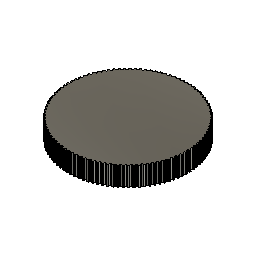
gear_99z (Autodesk Fusion 360 design; units mm, degrees)
Autodesk Fusion 360 part; units mm, degrees
sketch "Sketch1" plane through (0, 0, 0) normal (0, 0, 1) x (1, 0, 0) in component "gt2 pulley"
  circle A0 centre (0, 0) radius 31.5127 construction
  circle A1 centre (0, 0) radius 30.5087 construction
  line L0 (0, 0) -> (0, 31.5127) construction
  line L1 (0, 0) -> (0.9998, 31.4968) construction
  line L2 (0, 0) -> (1.4041, 31.4814) construction
  circle A2 centre (0, 0) radius 31.2587 construction
  arc A3 (0.3982, 31.1233) -> (0.4778, 30.824) centre (1.3927, 31.2276) ccw
  circle A4 centre (0, 0) radius 31.1087 construction
  arc A5 (0.2501, 31.2577) -> (0, 31.2587) centre (0, 0) ccw
  arc A6 (0.3982, 31.1233) -> (0.2501, 31.2577) centre (0.249, 31.1077) ccw
  arc A7 (0.4778, 30.824) -> (0.968, 30.4933) centre (0.9856, 31.048) ccw
  arc A8 (0, 31.2587) -> (-0.2501, 31.2577) centre (0, 0) ccw
  arc A9 (-0.2501, 31.2577) -> (-0.3982, 31.1233) centre (-0.249, 31.1077) ccw
  arc A10 (-0.4778, 30.824) -> (-0.3982, 31.1233) centre (-1.3927, 31.2276) ccw
  arc A11 (-0.9678, 30.4933) -> (-0.4778, 30.824) centre (-0.9856, 31.048) ccw
  arc A12 (0.968, 30.4933) -> (-0.968, 30.4933) centre (0, 0) ccw
  point P0 (1.3927, 31.2276)
  point P1 (0, 31.2587)
  dimension "d18" = 63.0254
  dimension "d19" = 1.818
  dimension "d22" = 1.004
  dimension "d24" = 0.75
  dimension "d26" = 1
  dimension "d27" = 0.15
  dimension "d28" = 0.15
  dimension "d47" = 0.555
  dimension "d52" = 3.812
  constraint coincident A0.centre A1.centre
  constraint coincident A0 L0.end
  constraint vertical L0
  constraint coincident A0 L1.end
  constraint coincident A0 L2.end
  constraint concentric A1 A2
  constraint coincident A1 A7.end
  constraint coincident L1 A7.end
  constraint coincident A2 P0
  constraint coincident L2 P0
  constraint coincident P0 A3.centre
  constraint coincident A2 P1
  constraint coincident L0 P1
  constraint concentric A2 A4
  constraint coincident P1 A5.end
  constraint coincident A4 A6.centre
  constraint coincident A3.start A6.start
  constraint tangent A3 A6
  constraint tangent A3 A7
  constraint symmetric L0 A7.end A12.end
  constraint symmetric L0 A3.start A9.end
  constraint symmetric L0 A3.end A10.start
  constraint symmetric L0 A3 A10
  constraint symmetric L0 A5.start A8.end
  constraint symmetric L0 P1 A5.end
  constraint symmetric L0 A5 A8
  constraint symmetric L0 A6 A9
  constraint symmetric L0 A7 A11
  constraint coincident A1 A11.start
  constraint tangent A1 A7
  constraint coincident L1 A7.centre
  measures "d18" diameter of A0
  measures "d19" angle of L0 L1
  measures "d22" distance of A0 A1
  measures "d24" distance of A1 A2
  measures "d26" radius of A3
  measures "d27" distance of A2 A4
  measures "d28" radius of A6
  measures "d47" radius of A7
extrude "Extrude1" add sketch "Sketch1" along normal blind 10 makes body 1
pattern_circular "C-Pattern1" count 99 over 360 about axis through (0, 0, 1.75) along (0, 0, 1) of bodies 1 makes body 2 at (-2.0422, 30.4402, 6.6667) makes body 3 at (-3.1141, 30.3493, 3.3333) makes body 4 at (-5.0327, 30.0907, 3.3333) makes body 5 at (-6.9311, 29.7109, 3.3333) makes body 6 at (-10.232, 28.7417, 6.6667) makes body 7 at (-11.4386, 28.2832, 6.6667) makes body 8 at (-13.7882, 27.2152, 6.6667) makes body 9 at (-14.1707, 27.0179, 3.3333) makes body 10 at (-17.1225, 25.2507, 6.6667) makes body 11 at (-17.477, 25.0067, 3.3333) makes body 12 at (-19.0278, 23.8479, 3.3333) makes body 13 at (-21.5918, 21.554, 6.6667) makes body 14 at (-21.8937, 21.2472, 6.6667) makes body 15 at (-23.1972, 19.8159, 3.3333) makes body 16 at (-24.9138, 17.6091, 6.6667) makes body 17 at (-26.2035, 15.6256, 6.6667) makes body 18 at (-26.5282, 15.0677, 3.3333) makes body 19 at (-27.7961, 12.5759, 6.6667) makes body 20 at (-28.5378, 10.7877, 6.6667) makes body 21 at (-28.9004, 9.7749, 3.3333) makes body 22 at (-29.4621, 7.9222, 3.3333) makes body 23 at (-30.0637, 5.1919, 6.6667) makes body 24 at (-30.3324, 3.2747, 6.6667) makes body 25 at (-30.429, 2.2033, 3.3333) makes body 26 at (-30.5029, -0.5915, 6.6667) makes body 27 at (-30.4631, -1.6665, 3.3333) makes body 28 at (-30.2961, -3.5952, 3.3333) makes body 29 at (-30.0071, -5.5095, 3.3333) makes body 30 at (-29.196, -8.8528, 6.6667) makes body 31 at (-29.0682, -9.2638, 3.3333) makes body 32 at (-28.4221, -11.0888, 3.3333) makes body 33 at (-26.993, -14.2182, 6.6667) makes body 34 at (-26.7897, -14.5976, 3.3333) makes body 35 at (-25.8099, -16.2673, 3.3333) makes body 36 at (-24.7262, -17.8716, 3.3333) makes body 37 at (-22.9864, -20.06, 6.6667) makes body 38 at (-22.2649, -20.8579, 3.3333) makes body 39 at (-20.262, -22.8086, 6.6667) makes body 40 at (-19.4453, -23.5087, 3.3333) makes body 41 at (-16.6749, -25.5485, 6.6667) makes body 42 at (-15.5793, -26.231, 6.6667) makes body 43 at (-13.8843, -27.1663, 6.6667) makes body 44 at (-12.9179, -27.6389, 3.3333) makes body 45 at (-9.724, -28.9175, 6.6667) makes body 46 at (-9.3151, -29.0518, 3.3333) makes body 47 at (-7.4538, -29.5841, 3.3333) makes body 48 at (-5.5624, -29.9973, 3.3333) makes body 49 at (-3.6487, -30.2897, 3.3333) makes body 50 at (-1.0756, -30.4897, 6.6667) makes body 51 at (0.2151, -30.5079, 3.3333) makes body 52 at (2.1496, -30.4329, 6.6667) makes body 53 at (4.7141, -30.1423, 6.6667) makes body 54 at (6.6163, -29.7826, 6.6667) makes body 55 at (9.315, -29.0519, 6.6667) makes body 56 at (10.5355, -28.6318, 6.6667) makes body 57 at (12.1332, -27.9922, 6.6667) makes body 58 at (14.6447, -26.764, 6.6667) makes body 59 at (15.0208, -26.5547, 3.3333) makes body 60 at (16.6748, -25.5486, 3.3333) makes body 61 at (19.4452, -23.5088, 6.6667) makes body 62 at (20.4222, -22.6652, 6.6667) makes body 63 at (21.2086, -21.9312, 3.3333) makes body 64 at (23.5429, -19.4039, 6.6667) makes body 65 at (23.8143, -19.0699, 3.3333) makes body 66 at (25.8099, -16.2675, 6.6667) makes body 67 at (26.7896, -14.5978, 6.6667) makes body 68 at (27.2876, -13.6442, 6.6667) makes body 69 at (28.1812, -11.6877, 6.6667) makes body 70 at (29.0682, -9.264, 6.6667) makes body 71 at (29.434, -8.0261, 6.6667) makes body 72 at (29.6987, -6.9835, 3.3333) makes body 73 at (30.2961, -3.5954, 6.6667) makes body 74 at (30.4211, -2.3107, 6.6667) makes body 75 at (30.5064, -0.3766, 6.6667) makes body 76 at (30.5007, 0.6991, 3.3333) makes body 77 at (30.3949, 2.6322, 3.3333) makes body 78 at (30.0263, 5.4036, 6.6667) makes body 79 at (29.6232, 7.2971, 6.6667) makes body 80 at (29.3475, 8.3369, 3.3333) makes body 81 at (28.4611, 10.9885, 6.6667) makes body 82 at (28.056, 11.985, 3.3333) makes body 83 at (26.5283, 15.0675, 6.6667) makes body 84 at (26.3131, 15.4403, 6.6667) makes body 85 at (24.7891, 17.7842, 6.6667) makes body 86 at (23.1973, 19.8157, 6.6667) makes body 87 at (22.9155, 20.141, 6.6667) makes body 88 at (21.5919, 21.5539, 3.3333) makes body 89 at (19.028, 23.8478, 6.6667) makes body 90 at (17.4771, 25.0066, 6.6667) makes body 91 at (17.1226, 25.2506, 3.3333) makes body 92 at (14.7392, 26.7121, 6.6667) makes body 93 at (13.7883, 27.2151, 3.3333) makes body 94 at (10.6366, 28.5944, 6.6667) makes body 95 at (10.2322, 28.7416, 3.3333) makes body 96 at (6.9312, 29.7109, 6.6667) makes body 97 at (5.0329, 30.0907, 6.6667) makes body 98 at (4.6079, 30.1587, 3.3333) makes body 99 at (2.6858, 30.3902, 3.3333)
sketch "Sketch2" plane through (0, 0, 10) normal (0, 0, 1) x (-1, 0, 0)
  arc A0 (-15.48, -27.0035) -> (-15.416, -27.1929) centre (-15.342, -27.0624) ccw
  arc A1 (-15.416, -27.1929) -> (-14.9788, -27.4361) centre (0, 0) ccw
  arc A2 (-14.9788, -27.4361) -> (-14.7841, -27.3907) centre (-14.9069, -27.3045) ccw
  arc A3 (-14.569, -27.1679) -> (-14.7841, -27.3907) centre (-13.9657, -27.9654) ccw
  arc A4 (-13.98, -27.1171) -> (-14.569, -27.1679) centre (-14.2342, -27.6105) ccw
  arc A5 (-15.6716, -26.1759) -> (-13.98, -27.1171) centre (0, 0) ccw
  arc A6 (-15.4041, -26.7033) -> (-15.6716, -26.1759) centre (-15.9567, -26.6521) ccw
  arc A7 (-15.48, -27.0035) -> (-15.4041, -26.7033) centre (-16.3998, -26.6111) ccw
  circle A8 centre (0, 0) radius 30.5087
  constraint coincident A1.centre A5.centre
extrude "Extrude2" add sketch "Sketch2" against normal blind 10 contours A5 A8 bodies 1 2 3 4 5 6 7 8 9 10 11 12 13 14 15 16 17 18 19 20 21 22 23 24 25 26 27 28 29 30 31 32 33 34 35 36 37 38 39 40 41 42 43 44 45 46 47 48 49 50 51 52 53 54 55 56 57 58 59 60 61 62 63 64 65 66 67 68 69 70 71 72 73 74 75 76 77 78 79 80 81 82 83 84 85 86 87 88 89 90 91 92 93 94 95 96 97 98 99
extrude "Extrude4" [suppressed] in component "gt2 pulley"
pattern_circular "C-Pattern7" [suppressed] in component "gt2 pulley"
extrude "Extrude3" [suppressed] in component "gt2 pulley"
pattern_circular "C-Pattern6" [suppressed] in component "gt2 pulley"
extrude "Extrude2'" [suppressed] in component "gt2 pulley"
pattern_circular "C-Pattern5" [suppressed] in component "gt2 pulley"
extrude "Extrude1'" [suppressed] in component "gt2 pulley"
pattern_circular "C-Pattern4" [suppressed] in component "gt2 pulley"
pattern_circular "C-Pattern3" [suppressed] in component "gt2 pulley"
pattern_circular "C-Pattern2" [suppressed] in component "gt2 pulley"
pattern_circular "C-Pattern1'" [suppressed] in component "gt2 pulley"
copy_body "Body->Comp1" [suppressed] in component "Component"
copy_body "Body->Comp2" [suppressed] in component "Component'"
copy_body "Body->Comp3" [suppressed] in component "Component''"
copy_body "Body->Comp4" [suppressed] in component "Component'''"
copy_body "Body->Comp5" [suppressed] in component "Component''''"
copy_body "Body->Comp6" [suppressed] in component "Component'''''"
copy_body "Body->Comp7" [suppressed] in component "Component''''''"
copy_body "Body->Comp8" [suppressed] in component "Component'''''''"
copy_body "Body->Comp9" [suppressed] in component "Component''''''''"
copy_body "Body->Comp10" [suppressed] in component "Component'''''''''"
copy_body "Body->Comp11" [suppressed] in component "Component''''''''''"
copy_body "Body->Comp12" [suppressed] in component "Component'''''''''''"
copy_body "Body->Comp13" [suppressed] in component "Component''''''''''''"
copy_body "Body->Comp14" [suppressed] in component "Component'''''''''''''"
copy_body "Body->Comp15" [suppressed] in component "Component''''''''''''''"
copy_body "Body->Comp16" [suppressed] in component "Component'''''''''''''''"
copy_body "Body->Comp17" [suppressed] in component "Component''''''''''''''''"
copy_body "Body->Comp18" [suppressed] in component "Component'''''''''''''''''"
copy_body "Body->Comp19" [suppressed] in component "Component''''''''''''''''''"
copy_body "Body->Comp20" [suppressed] in component "Component'''''''''''''''''''"
component "gt2 pulley" placed x (1, 0, 0) y (0, 1, 0) z (0, 0, 1) at (0, 0, 0)
equation "NumTeeth = 99" comment "min 20"
equation "ToothPitch = 2 mm"
equation "PullyDia = NumTeeth * ToothPitch / PI"
equation "ToothAng = ( ( 360 / NumTeeth ) * 1 deg )"
equation "TransOffsetAngle = ToothAng * 0.2"
equation "Sholulder_Radius = 0.15 mm"
equation "Root_Radius = 0.555 mm"
equation "TransRadius = 1 mm"
equation "ToolHeight = 0.75 mm"
equation "PLD = 0.254 mm"
equation "d18 = PullyDia"
equation "d19 = ToothAng / 2"
equation "d22 = PLD + ToolHeight"
equation "d24 = ToolHeight"
equation "d26 = TransRadius"
equation "d27 = Sholulder_Radius"
equation "d31 = NumTeeth"
equation "d33 = NumTeeth"
equation "d35 = NumTeeth"
equation "d37 = NumTeeth"
equation "d41 = NumTeeth"
equation "d45 = NumTeeth"
equation "d47 = Root_Radius"
equation "d50 = NumTeeth"
